Autodesk Fusion 360 part; units mm, degrees
(part 2 of 2)
sketch "Sketch1" plane through (0, 0, 0) normal (0, 0, 1) x (1, 0, 0)
  circle A0 centre (0, 0) radius 70
  line L0 (11.5, 29) -> (-11.5, 29) construction
  line L1 (-11.5, 29) -> (-11.5, -29) construction
  line L2 (-11.5, -29) -> (11.5, -29) construction
  line L3 (11.5, -29) -> (11.5, 29) construction
  line L4 (11.5, 29) -> (-11.5, -29) construction
  line L5 (-11.5, 29) -> (11.5, -29) construction
  circle A1 centre (11.5, 29) radius 1.5
  line L6 (0, 29) -> (0, -29) construction
  line L7 (-49.25, 0) -> (49.25, 0) construction
  circle A2 centre (-11.5, 29) radius 1.5
  circle A3 centre (-11.5, -29) radius 1.5
  circle A4 centre (11.5, -29) radius 1.5
  circle A5 centre (-49.25, -12.25) radius 1.5
  circle A6 centre (49.25, 0) radius 1.5
  line L8 (48, 22.5) -> (-48, 22.5) construction
  line L9 (-48, 22.5) -> (-48, -22.5) construction
  line L10 (-48, -22.5) -> (48, -22.5) construction
  line L11 (48, -22.5) -> (48, 22.5) construction
  line L12 (48, 22.5) -> (-48, -22.5) construction
  line L13 (-48, 22.5) -> (48, -22.5) construction
  line L14 (15, 32.5) -> (-15, 32.5) construction
  line L15 (-15, 32.5) -> (-15, -32.5) construction
  line L16 (-15, -32.5) -> (15, -32.5) construction
  line L17 (15, -32.5) -> (15, 32.5) construction
  line L18 (15, 32.5) -> (-15, -32.5) construction
  line L19 (-15, 32.5) -> (15, -32.5) construction
  line L20 (-20, -30.5) -> (-42, -30.5)
  line L21 (-42, -30.5) -> (-42, -22.5)
  line L22 (-42, -22.5) -> (-20, -22.5)
  line L23 (-20, -22.5) -> (-20, -30.5)
  line L24 (-20, -30.5) -> (-42, -22.5) construction
  line L25 (-42, -30.5) -> (-20, -22.5) construction
  line L26 (20, -22.5) -> (20, -30.5)
  line L27 (20, -30.5) -> (42, -30.5)
  line L28 (42, -30.5) -> (42, -22.5)
  line L29 (20, -30.5) -> (42, -22.5) construction
  line L30 (42, -30.5) -> (20, -22.5) construction
  line L31 (20, -22.5) -> (42, -22.5)
  line L32 (-42, 30.5) -> (-42, 22.5)
  line L33 (-20, 30.5) -> (-42, 30.5)
  line L34 (-20, 22.5) -> (-20, 30.5)
  line L35 (20, 30.5) -> (42, 30.5)
  line L36 (20, 30.5) -> (42, 22.5) construction
  line L37 (20, 22.5) -> (20, 30.5)
  line L38 (42, 30.5) -> (20, 22.5) construction
  line L39 (42, 30.5) -> (42, 22.5)
  line L40 (-42, 30.5) -> (-20, 22.5) construction
  line L41 (-20, 30.5) -> (-42, 22.5) construction
  line L42 (-42, 22.5) -> (-20, 22.5)
  line L43 (20, 22.5) -> (42, 22.5)
  circle A7 centre (-49.25, 12.25) radius 1.5
  line L44 (0, 70) -> (0, 65) construction
  line L45 (0, 65) -> (2, 65)
  line L46 (2, 65) -> (2, 69.9714)
  line L47 (-2, 65) -> (-2, 69.9714)
  line L48 (0, 65) -> (-2, 65)
  line L49 (-9, 25) -> (-13.5, 25)
  line L50 (-13.5, 25) -> (-13.5, -25)
  line L51 (-13.5, -25) -> (-9, -25)
  line L52 (-9, -25) -> (-9, 25)
  line L53 (-9, 25) -> (-13.5, -25) construction
  line L54 (-13.5, 25) -> (-9, -25) construction
  point P0 (-31, -26.5)
  point P1 (31, -26.5)
  point P2 (31, 26.5)
  point P3 (-31, 26.5)
  point P4 (-11.25, 0)
  dimension "d1" = 140
  dimension "d4" = 3
  dimension "d9" = 3
  dimension "d12" = 45
  dimension "d13" = 96
  dimension "d16" = 23
  dimension "d17" = 30
  dimension "d18" = 58
  dimension "d19" = 65
  dimension "d24" = 22
  dimension "d25" = 8
  dimension "d29" = 5
  dimension "d30" = 2
  dimension "d33" = 10.25
  dimension "d36" = 1.25
  dimension "d37" = 1.25
  dimension "d38" = 3
  dimension "d39" = 5
  dimension "d40" = 4
  dimension "d41" = 4.5
  dimension "d42" = 50
  dimension "d44" = 1.5
  constraint coincident A0.centre origin
  constraint perpendicular L0 L1
  constraint parallel L0 L2
  constraint parallel L1 L3
  constraint horizontal L0
  constraint coincident L4 A0.centre
  constraint coincident L5 A0.centre
  constraint coincident L0.start L3.end
  constraint midpoint L0 L6.start
  constraint midpoint L2 L6.end
  constraint symmetric A1 L6 A2
  constraint symmetric A1 L7 A4
  constraint symmetric L7 A2 A3
  constraint horizontal L7
  constraint midpoint A0.centre L7
  constraint perpendicular L8 L9
  constraint parallel L8 L10
  constraint parallel L9 L11
  constraint horizontal L8
  constraint coincident L12 A0.centre
  constraint coincident L13 A0.centre
  constraint perpendicular L14 L15
  constraint parallel L14 L16
  constraint parallel L15 L17
  constraint horizontal L14
  constraint coincident L18 A0.centre
  constraint coincident L19 A0.centre
  constraint perpendicular L20 L21
  constraint parallel L20 L22
  constraint parallel L21 L23
  constraint horizontal L20
  constraint coincident L24 P0
  constraint coincident L25 P0
  constraint symmetric L6 L20.start L26.end
  constraint symmetric L6 L20.end L27.end
  constraint symmetric L6 L21.end L28.end
  constraint symmetric L6 L22.end L26.start
  constraint symmetric L6 P0 P1
  constraint symmetric L7 L20.start L33.start
  constraint symmetric L7 L20.end L32.start
  constraint symmetric L7 L21.end L32.end
  constraint symmetric L7 L22.end L34.start
  constraint symmetric L7 P0 P3
  constraint symmetric L7 P1 P2
  constraint symmetric L7 L26.start L37.start
  constraint symmetric L7 L26.end L35.start
  constraint symmetric L7 L27.end L35.end
  constraint symmetric L7 L28.end L36.end
  constraint coincident L7.end A6.centre
  constraint symmetric L7 A5 A7
  constraint coincident A0 L44.start
  constraint vertical L44
  constraint perpendicular L44 L45
  constraint coincident A0 L46.end
  constraint perpendicular L45 L46
  constraint symmetric L45.start L44 L48.start
  constraint symmetric L44 L45.end L47.start
  constraint symmetric L44 L46.end L47.end
  constraint collinear A0.centre L44.start L44.end
  constraint perpendicular L49 L50
  constraint parallel L49 L51
  constraint parallel L50 L52
  constraint horizontal L49
  constraint coincident L53 P4
  constraint coincident L54 P4
  constraint coincident L7 P4
  measures "d1" diameter of A0
  measures "d4" diameter of A1
  measures "d9" diameter of A5
  measures "d12" distance of L8.end L9.end
  measures "d13" distance of L9.end L10.end
  measures "d16" distance of L1.end L2.end
  measures "d17" distance of L15.end L16.end
  measures "d18" distance of L0.end L1.end
  measures "d19" distance of L14.end L15.end
  measures "d24" distance of L20.start L20.end
  measures "d25" distance of L20.start L22.end A0.centre
  measures "d33" vertical distance of A5.centre L9.end
  measures "d36" distance of A5.centre L9
  measures "d37" distance of L7.end L11
  measures "d38" diameter of A6
  measures "d39" distance of L44.start L44.end
  measures "d40" distance of L45.end L47.start
  measures "d41" distance of L49.start L49.end
  measures "d42" distance of L49.end L50.end
  measures "d44" distance of L15 L50
extrude "Extrude1" add sketch "Sketch1" along normal blind 3 contours A0 L45 L46 L47 L48 | L49 L50 L51 L52 picked at (0.6667, -7.5)
sketch "Sketch2" plane through (0, 0, 3) normal (0, 0, 1) x (-1, 0, 0)
  line L0 (-42, 30.5) -> (-20, 30.5)
  line L1 (-20, 30.5) -> (-20, 22.5)
  line L2 (-20, 22.5) -> (-42, 22.5)
  line L3 (-42, 22.5) -> (-42, 30.5)
  line L4 (-20, -22.5) -> (-20, -30.5)
  line L5 (-20, -30.5) -> (-42, -30.5)
  line L6 (-42, -30.5) -> (-42, -22.5)
  line L7 (-42, -22.5) -> (-20, -22.5)
  circle A0 centre (49.25, -12.25) radius 1.5
  line L8 (20, -22.5) -> (42, -22.5)
  line L9 (42, -22.5) -> (42, -30.5)
  line L10 (42, -30.5) -> (20, -30.5)
  line L11 (20, -30.5) -> (20, -22.5)
  circle A1 centre (-11.5, 29) radius 1.5
  circle A2 centre (11.5, -29) radius 1.5
  circle A3 centre (-11.5, -29) radius 1.5
  circle A4 centre (11.5, 29) radius 1.5
  circle A5 centre (49.25, 12.25) radius 1.5
  circle A6 centre (-49.25, 0) radius 1.5
  line L12 (42, 22.5) -> (20, 22.5)
  line L13 (20, 22.5) -> (20, 30.5)
  line L14 (20, 30.5) -> (42, 30.5)
  line L15 (42, 30.5) -> (42, 22.5)
  line L16 (-2, -65) -> (2, -65)
  line L17 (2, -65) -> (2, -69.9714)
  arc A7 (2, -69.9714) -> (-2, -69.9714) centre (0, 0) ccw
  line L18 (-2, -69.9714) -> (-2, -65)
  line L19 (0, -25) -> (0, 0) construction
  line L20 (0, 0) -> (15, 0) construction
  line L21 (9, -25) -> (13.5, -25)
  line L22 (13.5, -25) -> (13.5, 25)
  line L23 (13.5, 25) -> (9, 25)
  line L24 (9, 25) -> (9, -25)
  line L25 (9, -25) -> (13.5, 25) construction
  line L26 (13.5, -25) -> (9, 25) construction
  point P0 (11.25, 0)
  dimension "d45" = 4.5
  dimension "d46" = 50
  dimension "d47" = 15
  dimension "d49" = 1.5
  constraint coincident A7.centre L19.end
  constraint perpendicular L10 L19
  constraint perpendicular L19 L20
  constraint perpendicular L21 L22
  constraint parallel L21 L23
  constraint parallel L22 L24
  constraint horizontal L21
  constraint coincident L25 P0
  constraint coincident L26 P0
  constraint coincident L20 P0
  constraint collinear L19.start L21.start L21.end
  measures "d45" distance of L21.start L21.end
  measures "d46" distance of L21.end L22.end
  measures "d47" distance of A7.centre L20.end
  measures "d49" distance of L20.end L22
extrude "Extrude2" cut sketch "Sketch2" against normal blind 1.5 contours L21 L22 L23 L24
